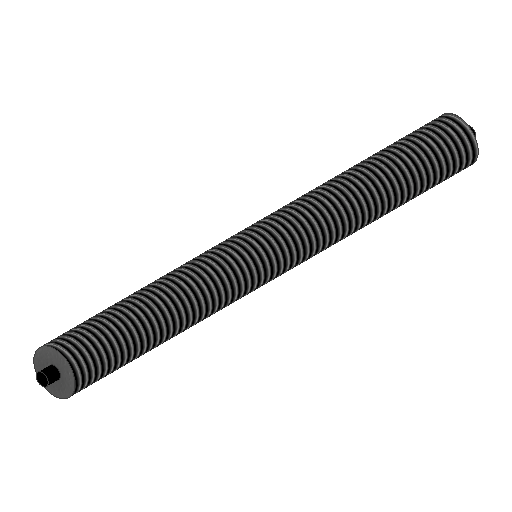
# Autodesk Inventor part: Coletor - Intake
Saved by Autodesk Inventor 2025.3 (Build 293356000, 356)
## iProperties
Created: 2026-05-13
Part Number: Coletor - Intake
Material: Genérico
Document SubType Name: Modeling
Designer: djair.oliveira
Density: 1 g/cm^3
Appearance: Padrão
Author: djair.oliveira
Autodesk Inventor part; units mm, degrees
ref_plane "YZ Plane" through (0, 0, 0) normal (1, 0, 0) x (0, 1, 0)
ref_plane "XZ Plane" through (0, 0, 0) normal (0, 1, 0) x (-1, 0, 0)
ref_plane "XY Plane" through (0, 0, 0) normal (0, 0, 1) x (1, 0, 0)
sketch "Esboço1" plane through (0, 0, 0) normal (1, 0, 0) x (0, 1, 0)
  line L0 (0, 0) -> (0, -525.4)
  line L1 (0, 0) -> (7.5, 0)
  line L2 (7.5, 0) -> (7.5, -525.4)
  line L3 (7.5, -525.4) -> (0, -525.4)
  line L4 (0, -525.4) -> (0, 0)
  line L5 (7.5, -15) -> (25.4, -15)
  line L6 (25.4, -15) -> (25.4, -510.4)
  line L7 (25.4, -510.4) -> (7.5, -510.4)
  line L8 (7.5, -510.4) -> (7.5, -15)
  point P0 (3.75, 0)
  point P1 (3.75, -525.4)
  point P2 (7.5, -510.4)
  dimension "d0" = 525.4
  dimension "d1" = 7.5
  dimension "d2" = 25.4
  dimension "d3" = 15
  dimension "d4" = 15
  constraints: 18 end point, 4 parallel, 2 horizontal, 2 midpoint, 2 perpendicular, 1 point on line, 1 vertical
  measures "d0" distance of L0.start L0.end
  measures "d1" distance of L2.end L3.end
  measures "d2" distance between parallel lines of L0 L6
  measures "d3" distance from line of point (3.75, 0) L5
  measures "d4" distance from line of point (3.75, -525.4) L7
revolve "Revolução1" add sketch "Esboço1" angle 360 about axis through (0, 0, -525.4) along (0, 0, 1)
thread "Rosca1" size "M1060x8" class "6g" standard "ANSI Metric M Profile" length 495.4
